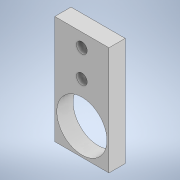
# Autodesk Inventor part: Button Panel
Saved by Autodesk Inventor 2022.1 (Build 261234000, 234)
## iProperties
Created: 2023-05-17
Part Number: Button Panel
Material: Generic
Document SubType Name: Modeling
Designer: brenden_deutschman
Density: 1 g/cm^3
Appearance: Default
Author: brenden_deutschman
Autodesk Inventor part; units mm, degrees
ref_plane "YZ Plane" through (0, 0, 0) normal (1, 0, 0) x (0, 1, 0)
ref_plane "XZ Plane" through (0, 0, 0) normal (0, 1, 0) x (-1, 0, 0)
ref_plane "XY Plane" through (0, 0, 0) normal (0, 0, 1) x (1, 0, 0)
sketch "Sketch1" plane through (0, 0, 0) normal (0, 0, 1) x (1, 0, 0)
  line L0 (12.7, -25.4) -> (-12.7, -25.4)
  line L1 (-12.7, -25.4) -> (-12.7, 25.4)
  line L2 (-12.7, 25.4) -> (12.7, 25.4)
  line L3 (12.7, 25.4) -> (12.7, -25.4)
  line L4 (12.7, -25.4) -> (-12.7, 25.4) construction
  line L5 (-12.7, -25.4) -> (12.7, 25.4) construction
  circle A0 centre (0, 6.35) radius 2.5
  circle A1 centre (0, 19.05) radius 2.5
  circle A2 centre (0, -12.7) radius 11.7475
  point P0 (0, 0)
  point P1 (0, 0)
  point P2 (0, 0)
  dimension "d0" = 25.4
  dimension "d1" = 50.8
  dimension "d2" = 5
  dimension "d3" = 5
  dimension "d4" = 12.7
  dimension "d5" = 6.35
  dimension "d6" = 19.05
  dimension "d7" = 23.495
  constraints: 12 end point, 4 midpoint, 3 centre point, 2 parallel, 1 horizontal, 1 perpendicular
  measures "d0" distance of L1.end L2.end
  measures "d1" distance of L0.end L1.end
  measures "d2" diameter of A0
  measures "d3" diameter of A1
  measures "d4" distance of A0.centre A1.centre
  measures "d5" distance of point (0, 0) A0.centre
  measures "d6" distance of point (0, 0) A1.centre
  measures "d7" diameter of A2
extrude "Extrusion1" add sketch "Sketch1" against normal blind 7.62
body "Solid1"
